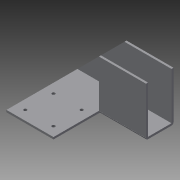
# Autodesk Inventor part: Arm holder Bracket
Saved by Autodesk Inventor 2015 (Build 190159000, 159)
## iProperties
Created: 2015-01-19
Part Number: Arm holder Bracket
Material: Generic
Document SubType Name: Modeling
Designer: chapale16
Density: 1 g/cm^3
Appearance: Default
Author: chapale16
Autodesk Inventor part; units mm, degrees
ref_plane "YZ Plane" through (0, 0, 0) normal (1, 0, 0) x (0, 1, 0)
ref_plane "XZ Plane" through (0, 0, 0) normal (0, 1, 0) x (-1, 0, 0)
ref_plane "XY Plane" through (0, 0, 0) normal (0, 0, 1) x (1, 0, 0)
sketch "Sketch1" plane through (0, 0, 0) normal (0, 1, 0) x (-1, 0, 0)
  line L0 (0, 0) -> (-50.8, 0)
  line L1 (-50.8, 0) -> (-50.8, -50.8)
  line L2 (-50.8, -50.8) -> (0, -50.8)
  line L3 (0, -50.8) -> (0, 0)
  line L4 (-50.8, 0) -> (-101.6, 0)
  line L5 (-101.6, 0) -> (-101.6, -25.4)
  line L6 (-101.6, -25.4) -> (-50.8, -25.4)
  line L7 (-50.8, -25.4) -> (-50.8, 0)
  line L8 (-50.8, 0) -> (-101.6, 0)
  line L9 (-101.6, 0) -> (-101.6, 2.2098)
  line L10 (-101.6, 2.2098) -> (-50.8, 2.2098)
  line L11 (-50.8, 2.2098) -> (-50.8, 0)
  dimension "d0" = 50.8
  dimension "d1" = 50.8
  dimension "d2" = 50.8
  dimension "d3" = 2.2098
  constraints: 24 end point, 6 parallel, 3 horizontal, 3 perpendicular, 1 point on line
  measures "d0" distance of L2.end L1.end
  measures "d1" distance of L1.end L0.end
  measures "d2" distance of L6.end L5.end
  measures "d3" distance of L8.end L9.end
extrude "Extrusion1" add sketch "Sketch1" against normal blind 2.2098
extrude "Extrusion2" add sketch "Sketch1" along normal blind 50.8 contours L4 L9 L10 L11
fillet "Fillet1" radius 2.2098 1 edges at (76.2, -2.2098, 2.2098)
sketch "Sketch2" plane through (0, 0, 0) normal (0, 1, 0) x (1, 0, 0)
  line L0 (50.8, 0) -> (101.6, 0) projected
  line L1 (101.6, 0) -> (101.6, 25.4) projected
  line L2 (101.6, 25.4) -> (50.8, 25.4) projected
  line L3 (50.8, 25.4) -> (50.8, 50.8) projected
  line L4 (50.8, 50.8) -> (0, 50.8) projected
  line L5 (0, 50.8) -> (0, 0) projected
  line L6 (0, 0) -> (50.8, 0) projected
  line L7 (10.1727, 10.1727) -> (40.6273, 10.1727)
  line L8 (40.6273, 10.1727) -> (40.6273, 40.6273)
  line L9 (40.6273, 40.6273) -> (10.1727, 40.6273)
  line L10 (10.1727, 40.6273) -> (10.1727, 10.1727)
  dimension "d9" = 30.4546
  dimension "d10" = 30.4546
  constraints: 8 end point, 4 coincident, 2 parallel, 1 horizontal, 1 perpendicular
  measures "d9" distance of L9.end L8.end
  measures "d10" distance of L8.end L7.end
hole "Hole1" at (10.1727, 0, -40.6273) at (10.1727, 0, -10.1727) at (40.6273, 0, -40.6273) at (40.6273, 0, -10.1727) direction (0, -1, 0) diameter 3.302 end through all
sketch "Sketch3" plane through (0, 0, 0) normal (0, 1, 0) x (1, 0, 0)
  line L0 (50.8, 0) -> (101.6, 0)
  line L1 (101.6, 0) -> (101.6, 33.655)
  line L2 (101.6, 33.655) -> (50.8, 33.655)
  line L3 (50.8, 33.655) -> (50.8, 0)
  line L4 (50.8, 33.655) -> (101.6, 33.655)
  line L5 (101.6, 33.655) -> (101.6, 59.055)
  line L6 (101.6, 59.055) -> (50.8, 59.055)
  line L7 (50.8, 59.055) -> (50.8, 33.655)
  point P0 (0, 0)
  dimension "d18" = 33.655
  dimension "d19" = 25.4
  constraints: 16 end point, 4 parallel, 2 horizontal, 2 perpendicular, 1 point on line
  measures "d18" distance of L1.end L0.end
  measures "d19" distance of L5.end L4.end
extrude "Extrusion3" cut sketch "Sketch3" against normal blind 25.4 contours L3 L2 L1 L0
extrude "Extrusion4" add sketch "Sketch3" against normal blind 2.2098 contours L7 L6 L5 L2
sketch "Sketch4" plane through (0, 50.8, 0) normal (0, 1, 0) x (1, 0, 0)
  point P0 (0, 0)
sketch "Sketch5" plane through (0, 50.8, 0) normal (0, 1, 0) x (1, 0, 0)
  line L0 (50.8, 0) -> (101.6, 0)
  line L1 (101.6, 0) -> (101.6, -2.2098)
  line L2 (101.6, -2.2098) -> (50.8, -2.2098)
  line L3 (50.8, -2.2098) -> (50.8, 0)
  point P0 (0, 0)
  constraints: 8 end point, 2 parallel, 1 horizontal, 1 perpendicular
extrude "Extrusion5" cut sketch "Sketch5" against normal through all
sketch "Sketch7" plane through (0, -2.2098, 0) normal (0, -1, 0) x (1, 0, 0)
  line L0 (50.8, -33.655) -> (101.6, -33.655)
  line L1 (101.6, -33.655) -> (101.6, -31.4452)
  line L2 (101.6, -31.4452) -> (50.8, -31.4452)
  line L3 (50.8, -31.4452) -> (50.8, -33.655)
  point P0 (0, 0)
  dimension "d27" = 50.8
  dimension "d28" = 2.2098
  constraints: 8 end point, 2 parallel, 1 horizontal, 1 perpendicular
  measures "d27" distance of L2.end L1.end
  measures "d28" distance of L1.end L0.end
extrude "Extrusion6" add sketch "Sketch7" against normal blind 53.0098
fillet "Fillet2" radius 2.2098 1 edges at (76.2, -2.2098, -31.4452)
sketch "Sketch8" plane through (0, 0, 0) normal (0, 1, 0) x (1, 0, 0)
  line L0 (50.8, 0) -> (50.8, 31.4452) projected
  line L1 (50.8, 31.4452) -> (50.8, 33.655) projected
  line L2 (50.8, 33.655) -> (101.6, 33.655) projected
  line L3 (101.6, 33.655) -> (101.6, 59.055) projected
  line L4 (101.6, 59.055) -> (50.8, 59.055) projected
  line L5 (50.8, 59.055) -> (50.8, 50.8) projected
  line L6 (50.8, 50.8) -> (0, 50.8) projected
  line L7 (0, 50.8) -> (0, 0) projected
  line L8 (0, 0) -> (50.8, 0) projected
  circle A0 centre (40.6273, 10.1727) radius 1.651 projected
  circle A1 centre (10.1727, 10.1727) radius 1.651 projected
  circle A2 centre (10.1727, 40.6273) radius 1.651 projected
  circle A3 centre (40.6273, 40.6273) radius 1.651 projected
  line L9 (50.8, 59.055) -> (101.6, 59.055)
  line L10 (101.6, 59.055) -> (101.6, 76.6318)
  line L11 (101.6, 76.6318) -> (50.8, 76.6318)
  line L12 (50.8, 76.6318) -> (50.8, 59.055)
  line L13 (50.8, 50.8) -> (0, 50.8)
  line L14 (0, 50.8) -> (0, 76.6318)
  line L15 (0, 76.6318) -> (50.8, 76.6318)
  line L16 (50.8, 76.6318) -> (50.8, 50.8)
  dimension "d32" = 17.5768
  constraints: 16 end point, 4 parallel, 2 horizontal, 2 perpendicular, 1 point on line
  measures "d32" distance of L10.end L9.end
extrude "Extrusion7" add sketch "Sketch8" against normal blind 2.2098 contours L14 L15 L12 L5 L6 | L4 L12 L11 L10
sketch "Sketch9" plane through (0, 0, 0) normal (0, 1, 0) x (1, 0, 0)
  line L0 (101.6, 76.6318) -> (50.8, 76.6318)
  line L1 (50.8, 76.6318) -> (50.8, 51.2318)
  line L2 (50.8, 51.2318) -> (101.6, 51.2318)
  line L3 (101.6, 51.2318) -> (101.6, 76.6318)
  line L4 (50.8, 51.2318) -> (112.668, 51.2318)
  line L5 (112.668, 51.2318) -> (112.668, 0)
  line L6 (112.668, 0) -> (50.8, 0)
  line L7 (50.8, 0) -> (50.8, 51.2318)
  point P0 (0, 0)
  dimension "d35" = 25.4
  constraints: 16 end point, 4 parallel, 2 horizontal, 2 perpendicular
  measures "d35" distance of L1.end L0.end
extrude "Extrusion8" cut sketch "Sketch9" against normal blind 2.2098 contours L4 L5 L6 L7 L2
sketch "Sketch10" plane through (0, 50.8, 0) normal (0, 1, 0) x (1, 0, 0)
  line L0 (50.8, 33.655) -> (116.0287, 33.655)
  line L1 (116.0287, 33.655) -> (116.0287, 19.3076)
  line L2 (116.0287, 19.3076) -> (50.8, 19.3076)
  line L3 (50.8, 19.3076) -> (50.8, 33.655)
  point P0 (0, 0)
  constraints: 8 end point, 2 parallel, 1 horizontal, 1 perpendicular
extrude "Extrusion9" cut sketch "Sketch10" against normal through all
sketch "Sketch11" plane through (0, 0, 0) normal (0, 1, 0) x (1, 0, 0)
  line L0 (50.8, 51.2318) -> (101.6, 51.2318) projected
  line L1 (101.6, 51.2318) -> (101.6, 76.6318) projected
  line L2 (101.6, 76.6318) -> (0, 76.6318) projected
  line L3 (0, 76.6318) -> (0, 0) projected
  line L4 (0, 0) -> (50.8, 0) projected
  line L5 (50.8, 0) -> (50.8, 51.2318) projected
  circle A0 centre (40.6273, 10.1727) radius 1.651 projected
  circle A1 centre (10.1727, 10.1727) radius 1.651 projected
  circle A2 centre (10.1727, 40.6273) radius 1.651 projected
  circle A3 centre (40.6273, 40.6273) radius 1.651 projected
  line L6 (50.8, 51.2318) -> (101.6, 51.2318)
  line L7 (101.6, 51.2318) -> (101.6, 49.022)
  line L8 (101.6, 49.022) -> (50.8, 49.022)
  line L9 (50.8, 49.022) -> (50.8, 51.2318)
  dimension "d40" = 2.2098
  constraints: 8 end point, 2 parallel, 1 horizontal, 1 perpendicular
  measures "d40" distance of L6.end L7.end
extrude "Extrusion10" add sketch "Sketch11" along normal blind 50.8 contours L0 L7 L8 L5
sketch "Sketch12" plane through (0, 0, 0) normal (0, -1, 0) x (1, 0, 0)
  line L0 (50.8, -51.2318) -> (50.8, -49.022) projected
  line L1 (101.6, -48.9148) -> (50.8, -48.9148)
  line L2 (50.8, -48.9148) -> (50.8, -51.1246)
  line L3 (50.8, -51.1246) -> (101.6, -51.1246)
  line L4 (101.6, -51.1246) -> (101.6, -48.9148)
  point P0 (0, 0)
  dimension "d43" = 2.2098
  constraints: 8 end point, 2 parallel, 1 horizontal, 1 perpendicular, 1 point on line
  measures "d43" distance of L2.end L1.end
extrude "Extrusion11" add sketch "Sketch12" along normal blind 2.2098
fillet "Fillet3" radius 2.2098 1 edges at (76.2, -2.2098, -48.9148)
sketch "Sketch14" plane through (0, -2.2098, 0) normal (0, -1, 0) x (1, 0, 0)
  line L0 (101.6, -76.6318) -> (0, -76.6318)
  line L1 (0, -76.6318) -> (0, -78.8416)
  line L2 (0, -78.8416) -> (101.6, -78.8416)
  line L3 (101.6, -78.8416) -> (101.6, -76.6318)
  point P0 (0, 0)
  dimension "d47" = 2.2098
  constraints: 8 end point, 2 parallel, 1 horizontal, 1 perpendicular
  measures "d47" distance of L1.end L0.end
extrude "Extrusion12" add sketch "Sketch14" against normal blind 53.0098
sketch "Sketch15" plane through (101.6, -2.2098, -78.8416) normal (0, 0, -1) x (-1, 0, 0)
  line L0 (101.6, 53.0098) -> (0, 53.0098) projected
  line L1 (101.6, 2.2098) -> (50.8, 53.0098)
  line L2 (101.6, 2.2098) -> (101.6, 53.0098)
  line L3 (101.6, 2.2098) -> (101.6, 53.0098) projected
  line L4 (101.6, 53.0098) -> (50.8, 53.0098)
  dimension "d50" = 50.8
  constraints: 6 end point, 1 collinear, 1 midpoint, 1 perpendicular
  measures "d50" distance of L0.end L1.end
extrude "Extrusion13" cut sketch "Sketch15" against normal blind 2.2098
fillet "Fillet4" radius 2.2098 1 edges at (50.8, -2.2098, -78.8416)
body "Solid1"
